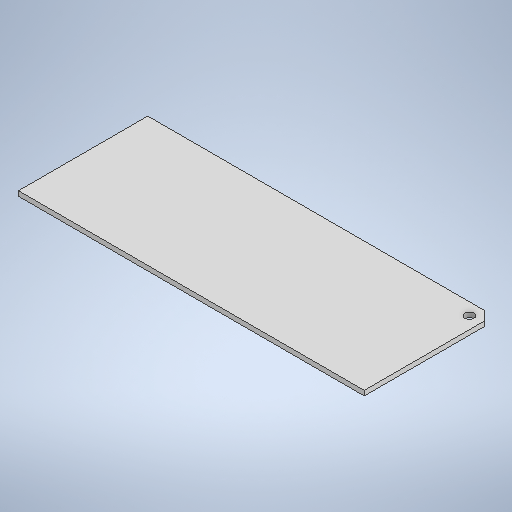
# Autodesk Inventor part: teaser_PCB
Saved by Autodesk Inventor 2025.2 (Build 292293000, 293)
## iProperties
Created: 2025-03-24
Part Number: teaser_PCB
Material: Generic
Document SubType Name: Modeling
Designer: Acer
Density: 1 g/cm^3
Appearance: Default
Author: Acer
Autodesk Inventor part; units mm, degrees
ref_plane "YZ Plane" through (0, 0, 0) normal (1, 0, 0) x (0, 1, 0)
ref_plane "XZ Plane" through (0, 0, 0) normal (0, 1, 0) x (-1, 0, 0)
ref_plane "XY Plane" through (0, 0, 0) normal (0, 0, 1) x (1, 0, 0)
sketch "Sketch1" plane through (0, 0, 0) normal (0, 1, 0) x (-1, 0, 0)
  line L0 (-57.5, 21.5) -> (57.5, 21.5)
  line L1 (57.5, 21.5) -> (57.5, -21.5)
  line L2 (57.5, -21.5) -> (-57.5, -21.5)
  line L3 (-57.5, -21.5) -> (-57.5, 21.5)
  line L4 (-57.5, 21.5) -> (57.5, -21.5) construction
  line L5 (57.5, 21.5) -> (-57.5, -21.5) construction
  point P0 (0, 0)
  dimension "d0" = 115
  dimension "d1" = 43
  constraints: 12 end point, 2 midpoint, 2 parallel, 1 horizontal, 1 perpendicular
  measures "d0" distance of L1.end L2.end
  measures "d1" distance of L0.end L1.end
extrude "Extrusion1" add sketch "Sketch1" along normal blind 1.6
sketch "Sketch2" plane through (0, 1.6, 0) normal (0, 1, 0) x (1, 0, 0)
  line L0 (57.5, 21.5) -> (-57.5, 21.5) projected
  line L1 (57.5, 21.5) -> (54.5, 21.5)
  line L2 (57.5, -21.5) -> (57.5, 21.5) projected
  line L3 (54.5, 21.5) -> (57.5, 21.5)
  line L4 (57.5, 21.5) -> (57.5, 18.5)
  line L5 (57.5, 18.5) -> (54.5, 21.5)
  point P0 (0, 0)
  dimension "d4" = 3
  dimension "d5" = 3
  constraints: 8 end point, 2 point on line, 1 perpendicular
  measures "d4" distance of L0.start L1.end
  measures "d5" distance of L0.start L4.end
extrude "Extrusion2" cut sketch "Sketch2" against normal blind 1.6
sketch "Sketch3" plane through (0, 1.6, 0) normal (0, 1, 0) x (1, 0, 0)
  line L0 (57.5, -21.5) -> (57.5, 18.5) projected
  circle A0 centre (53.5, 17.5) radius 1.5
  point P0 (0, 0)
  dimension "d11" = 3
  constraints: 1 centre point
  measures "d11" diameter of A0
extrude "Extrusion3" cut sketch "Sketch3" against normal blind 1.6
body "Solid1"
